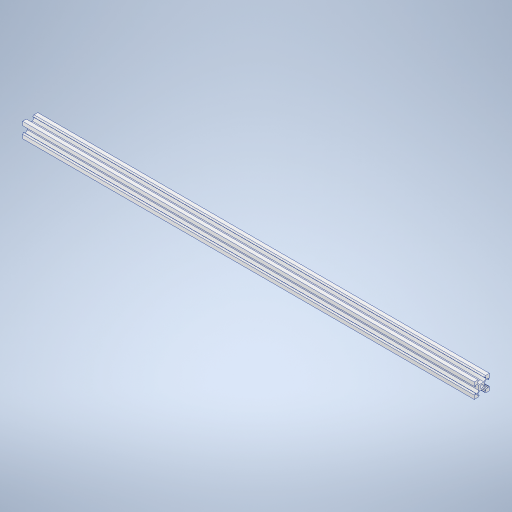
# Autodesk Inventor part: VSlot Extrusion 20x20x650mm
Saved by Autodesk Inventor 2023 (Build 270158000, 158)
## iProperties
Created: 2023-04-10
Part Number: VSlot Extrusion 20x20x650mm
Material: Aluminum 6061
Document SubType Name: Modeling
Designer: ethan
Density: 2.7 g/cm^3
Appearance: Aluminum - Flat
Author: ethan
Autodesk Inventor part; units mm, degrees
ref_plane "YZ Plane" through (0, 0, 0) normal (1, 0, 0) x (0, 1, 0)
ref_plane "XZ Plane" through (0, 0, 0) normal (0, 1, 0) x (-1, 0, 0)
sketch "Sketch1" plane through (0, 0, 0) normal (1, 0, 0) x (0, 1, 0)
  arc A0 (0, -2.15) -> (2.15, 0) centre (0, 0) ccw
  line L0 (3.75, 0) -> (3.75, -2.8308)
  line L1 (2.8308, -3.75) -> (0, -3.75)
  line L2 (0, 0) -> (10, 0) construction
  line L3 (10, 0) -> (10, -10) construction
  line L4 (10, -10) -> (0, -10) construction
  line L5 (0, -10) -> (0, 0) construction
  line L6 (3.75, -2.8308) -> (6.4192, -5.5)
  line L7 (2.8308, -3.75) -> (5.5, -6.4192)
  line L8 (5.5, -6.4192) -> (5.5, -8.2)
  line L9 (5.5, -8.2) -> (3.15, -8.2)
  line L10 (0, 0) -> (5.5, 0) construction
  line L11 (5.5, 0) -> (5.5, -5.5) construction
  line L12 (5.5, -5.5) -> (0, -5.5) construction
  line L13 (0, -5.5) -> (0, 0) construction
  line L14 (6.4192, -5.5) -> (8.2, -5.5)
  line L15 (3.4914, -8.5414) -> (4.95, -10)
  line L16 (3.6328, -8.2) -> (5.6956, -8.2) construction
  line L17 (8.2, -5.5) -> (8.2, -3.6328)
  line L18 (8.5414, -3.4914) -> (10, -4.95)
  line L19 (10, -4.95) -> (10, -10)
  line L20 (4.95, -10) -> (10, -10)
  arc A1 (2.15, 0) -> (0, -2.15) centre (0, 0) ccw construction
  arc A2 (3.6328, -8.2) -> (3.4914, -8.5414) centre (3.6328, -8.4) ccw
  arc A3 (8.5414, -3.4914) -> (8.2, -3.6328) centre (8.4, -3.6328) ccw
  line L21 (3.75, 0) -> (2.15, 0)
  line L22 (0, -2.15) -> (0, -3.75)
  point P0 (8.2, -3.15)
  dimension "d0" = 4.3
  dimension "d1" = 3.75
  dimension "d2" = 3.75
  dimension "d5" = 10
  dimension "d6" = 10
  dimension "d10" = 5.5
  dimension "d11" = 5.5
  dimension "d12" = 1.8
  dimension "d14" = 1.3
  dimension "d15" = 45
  dimension "d16" = 3.15
  dimension "d17" = 45
  dimension "d18" = 3.15
  dimension "d19" = 1.8
  dimension "d20" = 0.2
  constraints: 46 end point, 10 point on line, 8 point on circle, 5 horizontal, 5 parallel, 5 perpendicular, 4 centre point, 4 collinear, 4 tangent, 3 equal length, 3 vertical, 1 coincident, 1 equal radius
  measures "d0" diameter of A0
  measures "d1" distance from line of point (0, 0) L0
  measures "d2" distance from line of point (0, 0) L1
  measures "d5" distance of L3.end L4.end
  measures "d6" distance of L2.end L3.end
  measures "d10" distance of L11.end L12.end
  measures "d11" distance of L10.end L11.end
  measures "d12" distance between parallel lines of L4 L9
  measures "d14" distance between parallel lines of L7 L6
  measures "d15" angle of L15 L16
  measures "d16" distance from line of L5 L9.end
  measures "d17" angle of L17 L18
  measures "d18" distance from line of L2 point (8.2, -3.15)
  measures "d19" distance between parallel lines of L19 L17
  measures "d20" radius of A2
extrude "Extrusion1" add sketch "Sketch1" along normal blind 597.1
pattern_circular "Circular Pattern1" count 4 over 360 about axis through (0, 0, 0) along (-1, 0, 0) of "Extrusion1"
ref_plane "Work Plane1" through (0, 4.95, 0) normal (0, 0, 1) x (1, 0, 0)
equation "\"d2\" = d1"
equation "\"d18\" = d16"
equation "\"d19\" = d12"
body "Solid1"
